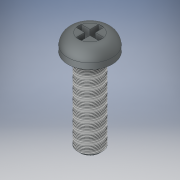
# Autodesk Inventor part: Screw
Saved by Autodesk Inventor 2017 (Build 210142000, 142)
## iProperties
Created: 2016-08-08
Part Number: Screw
Material: Generic
Document SubType Name: Modeling
Designer: ge937963
Density: 1 g/cm^3
Appearance: Zinc
Mass: 0.0509935 g
Surface Area: 1.10999 cm^2
Volume: 0.0509935 cm^3
Author: ge937963
Autodesk Inventor part; units mm, degrees
ref_plane "YZ Plane" through (0, 0, 0) normal (1, 0, 0) x (0, 1, 0)
ref_plane "XZ Plane" through (0, 0, 0) normal (0, 1, 0) x (-1, 0, 0)
ref_plane "XY Plane" through (0, 0, 0) normal (0, 0, 1) x (1, 0, 0)
sketch "Sketch1" plane through (0, 0, 0) normal (0, 1, 0) x (-1, 0, 0)
  circle A0 centre (0, 0) radius 1.1684
  dimension "d0" = 2.3368
  constraints: 1 centre point, 1 coincident
  measures "d0" diameter of A0
extrude "Extrusion1" add sketch "Sketch1" along normal blind 7.9375
sketch "Sketch2" plane through (0, 7.9375, 0) normal (0, 1, 0) x (1, 0, 0)
  circle A0 centre (0, 0) radius 1.1684 projected
  circle A1 centre (0, 0) radius 2.1209
  dimension "d3" = 4.2418
  constraints: 1 centre point, 1 coincident
  measures "d3" diameter of A1
extrude "Extrusion2" add sketch "Sketch2" along normal blind 1.5748 contours A0 | A1
fillet "Fillet1" radius 1.016 1 edges at (-2.1209, 9.5123, 0)
thread "Thread1" size "3-28" class "2B" standard "Inch Tapping Threads" full length
chamfer "Chamfer1" distance 0.254 angle 45 1 edges at (1.1684, 0, 0)
sketch "Sketch3" plane through (0, 9.5123, 0) normal (0, 1, 0) x (1, 0, 0)
  circle A0 centre (0, 0) radius 1.1049 projected
  line L0 (-0.254, -1.0753) -> (0.254, -1.0753)
  line L1 (0.254, -1.0753) -> (0.254, 1.0753)
  line L2 (0.254, 1.0753) -> (-0.254, 1.0753)
  line L3 (-0.254, 1.0753) -> (-0.254, -1.0753)
  line L4 (-1.0753, -0.254) -> (1.0753, -0.254)
  line L5 (1.0753, -0.254) -> (1.0753, 0.254)
  line L6 (1.0753, 0.254) -> (-1.0753, 0.254)
  line L7 (-1.0753, 0.254) -> (-1.0753, -0.254)
  point P0 (0, 1.0753)
  point P1 (1.0753, 0)
  dimension "d12" = 0.508
  constraints: 16 end point, 4 parallel, 4 perpendicular, 3 point on circle, 2 horizontal, 2 midpoint, 1 horizontal alignment, 1 vertical alignment
  measures "d12" distance of L6.end L4.start
extrude "Extrusion3" cut sketch "Sketch3" against normal blind 1.27 contours L5 L4 L1 L6 | L1 L6 L3 L2 | L1 L4 L3 L6 | L0 L3 L4 L1 | L3 L4 L7 L6
body "Solid1"
